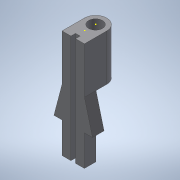
# Autodesk Inventor part: NO_GO_ZONE_2019_2020_DEVELOPMENT_CLASS
Saved by Autodesk Inventor 2020 (Build 240168000, 168)
## iProperties
Created: 2016-08-03
Part Number: NO_GO_ZONE_2019_2020_DEVELOPMENT_CLASS
Material: Generic
Document SubType Name: Modeling
Designer: Jon Fagg
Density: 1 g/cm^3
Appearance: Default
Author: Jon Fagg
Autodesk Inventor part; units mm, degrees
ref_plane "YZ Plane" through (0, 0, 0) normal (1, 0, 0) x (0, 1, 0)
ref_plane "XZ Plane" through (0, 0, 0) normal (0, 1, 0) x (-1, 0, 0)
ref_plane "XY Plane" through (0, 0, 0) normal (0, 0, 1) x (1, 0, 0)
sketch "Sketch1" plane through (0, 0, 0) normal (0, 0, 1) x (1, 0, 0)
  circle A0 centre (0, 0) radius 9
  line L0 (0, 0) -> (0, -29) construction
  line L1 (0, -29) -> (-3, -29) construction
  line L2 (3, -29) -> (0, -29) construction
  circle A1 centre (0, 0) radius 14.5
  line L3 (-14.5, 0) -> (-14.5, -29)
  line L4 (-14.5, -29) -> (-3, -29)
  line L5 (14.5, 0) -> (14.5, -29)
  line L6 (14.5, -29) -> (3, -29)
  line L7 (-3, -29) -> (-3, -23)
  line L8 (3, -29) -> (3, -23)
  line L9 (3, -23) -> (-3, -23)
  dimension "d0" = 18
  dimension "d1" = 29
  dimension "d2" = 3
  dimension "d4" = 5.5
  dimension "d5" = 6
  dimension "d6" = 6
  dimension "d7" = 3
  constraints: 20 end point, 5 vertical, 2 centre point, 2 perpendicular, 2 point on circle, 2 tangent, 1 coincident, 1 collinear, 1 horizontal, 1 point on line
  measures "d0" diameter of A0
  measures "d1" distance of L0.start L0.end
  measures "d2" distance of L0.end L1.end
  measures "d4" radial gap between concentric circles of A0 A1
  measures "d5" distance of L4.end L7.end
  measures "d6" distance of L8.end L7.end
  measures "d7" distance of L2.start L0.end
extrude "Extrusion1" add sketch "Sketch1" against normal blind 60 contours A0 | A1 | L5 L6 L8 L9 L7 L4 L3 A1
sketch "Sketch2" plane through (0, 0, 0) normal (0, 0, 1) x (1, 0, 0)
  circle A0 centre (0, 0) radius 9
  dimension "d10" = 18
  constraints: 1 centre point, 1 coincident
  measures "d10" diameter of A0
extrude "Extrusion2" cut sketch "Sketch2" against normal blind 52
sketch "Sketch3" plane through (0, 0, -60) normal (0, 0, -1) x (-1, 0, 0)
  line L0 (-3, -29) -> (-25, -29)
  line L1 (-25, -29) -> (-25, -14)
  line L2 (3, -29) -> (25, -29)
  line L3 (25, -29) -> (25, -14)
  line L4 (25, -14) -> (-25, -14)
  line L5 (-3, -29) -> (-3, -23)
  line L6 (-3, -23) -> (-3, -29) projected
  line L7 (-3, -23) -> (3, -23)
  line L8 (3, -23) -> (-3, -23) projected
  line L9 (3, -23) -> (3, -29)
  line L10 (3, -29) -> (3, -23) projected
  point P0 (0, 0)
  dimension "d13" = 22
  dimension "d14" = 15
  dimension "d15" = 22
  constraints: 16 end point, 3 collinear, 3 perpendicular, 2 horizontal
  measures "d13" distance of L0.start L0.end
  measures "d14" distance of L0.end L1.end
  measures "d15" distance of L2.start L2.end
extrude "Extrusion3" add sketch "Sketch3" against normal blind 20 and the other way blind 40
sketch "Sketch4" plane through (0, 0, -100) normal (0, 0, -1) x (-1, 0, 0)
  line L0 (-3, -29) -> (-14.5, -29)
  line L1 (-3, -29) -> (-14.5, -29) projected
  line L2 (-14.5, -29) -> (-14.5, -14)
  line L3 (-14.5, -29) -> (-14.5, -14) projected
  line L4 (-14.5, -14) -> (14.5, -14)
  line L5 (14.5, -14) -> (14.5, -29)
  line L6 (14.5, -14) -> (14.5, -29) projected
  line L7 (14.5, -29) -> (3, -29)
  line L8 (14.5, -29) -> (3, -29) projected
  line L9 (3, -29) -> (3, -23)
  line L10 (3, -29) -> (3, -23) projected
  line L11 (3, -23) -> (-3, -23)
  line L12 (3, -23) -> (-3, -23) projected
  line L13 (-3, -23) -> (-3, -29)
  line L14 (-3, -23) -> (-3, -29) projected
  point P0 (0, 0)
  constraints: 16 end point, 7 collinear, 1 perpendicular
extrude "Extrusion4" add sketch "Sketch4" along normal blind 40
sketch "Sketch5" plane through (0, 0, 0) normal (0, 0, 1) x (1, 0, 0)
  point P0 (0, 0)
sketch "Sketch6" plane through (0, 0, 0) normal (0, 0, 1) x (1, 0, 0)
  point P0 (0, 0)
sketch "Sketch7" plane through (-14.5, -14, -60) normal (0, 1, 0) x (1, 0, 0)
  line L0 (29, 0) -> (39.5, 40)
  line L1 (39.5, 40) -> (46.8581, 40)
  line L2 (39.5, -20) -> (39.5, 40) projected
  line L3 (46.8581, 40) -> (46.8581, -22.6176)
  line L4 (46.8581, -22.6176) -> (29, -22.6176)
  line L5 (29, -60) -> (29, -20) projected
  line L6 (29, 0) -> (29, -22.6176)
  point P0 (14.5, -60)
  constraints: 10 end point, 3 perpendicular, 1 collinear, 1 point on line
sketch "Sketch8" plane through (-14.5, -14, -60) normal (0, 1, 0) x (1, 0, 0)
  point P0 (14.5, -60)
extrude "Extrusion5" cut sketch "Sketch7" against normal blind 21.25
sketch "Sketch9" plane through (-25, -14, -40) normal (0, 1, 0) x (1, 0, 0)
  line L0 (0, 60) -> (10.5, 20)
  line L1 (10.5, 20) -> (10.5, -3.0244)
  line L2 (10.5, -3.0244) -> (-2.3194, -3.0244)
  line L3 (-2.3194, -3.0244) -> (-2.3194, 60)
  line L4 (-2.3194, 60) -> (0, 60)
  point P0 (25, -40)
  constraints: 10 end point, 2 perpendicular, 2 vertical
extrude "Extrusion6" cut sketch "Sketch9" against normal blind 22.5
sketch "Sketch10" plane through (0, 0, 0) normal (0, 0, 1) x (1, 0, 0)
  point P0 (0, 0)
body "Solid1"
